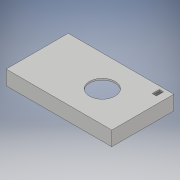
# Autodesk Inventor part: carrier_cmount
Saved by Autodesk Inventor 2018 (Build 220112000, 112)
## iProperties
Created: 2018-07-23
Part Number: carrier_cmount
Material: Generic
Document SubType Name: Modeling
Designer: matth
Density: 1 g/cm^3
Appearance: Default
Author: matth
Autodesk Inventor part; units mm, degrees
ref_plane "YZ Plane" through (0, 0, 0) normal (1, 0, 0) x (0, 1, 0)
ref_plane "XZ Plane" through (0, 0, 0) normal (0, 1, 0) x (-1, 0, 0)
ref_plane "XY Plane" through (0, 0, 0) normal (0, 0, 1) x (1, 0, 0)
sketch "Sketch1" plane through (0, 0, 0) normal (0, 0, 1) x (1, 0, 0)
  line L0 (-5.688, 3.2706) -> (94.312, 3.2706)
  line L1 (94.312, 3.2706) -> (94.312, -54.2294)
  line L2 (94.312, -54.2294) -> (-5.688, -54.2294)
  line L3 (-5.688, -54.2294) -> (-5.688, 3.2706)
  line L4 (95.812, 4.7706) -> (-7.188, 4.7706)
  line L5 (-7.188, 4.7706) -> (-7.188, -55.7294)
  line L6 (-7.188, -55.7294) -> (95.812, -55.7294)
  line L7 (95.812, -55.7294) -> (95.812, 4.7706)
  circle A0 centre (56.312, -25.4794) radius 12.5
  point P0 (0, 0)
  dimension "d0" = 100
  dimension "d1" = 57.5
  dimension "d2" = 1.5
  dimension "d3" = 25
  dimension "d4" = 38
  constraints: 16 end point, 4 parallel, 2 perpendicular, 1 centre point, 1 horizontal, 3 other
  measures "d0" distance of L1.end L2.end
  measures "d1" distance of L0.end L1.end
  measures "d2" distance between parallel lines of L0 L4
  measures "d3" diameter of A0
  measures "d4" distance from line of L1 A0.centre
extrude "Extrusion1" add sketch "Sketch1" along normal blind 1.5 contours L0 L1 L2 L3 | L7 L6 L5 L4
sketch "Sketch2" plane through (0, 0, 1.5) normal (0, 0, 1) x (1, 0, 0)
  line L0 (95.812, 4.7706) -> (-7.188, 4.7706) projected
  line L1 (-7.188, 4.7706) -> (-7.188, -55.7294) projected
  line L2 (-7.188, -55.7294) -> (95.812, -55.7294) projected
  line L3 (95.812, -55.7294) -> (95.812, 4.7706) projected
  line L4 (-5.688, 3.2706) -> (94.312, 3.2706)
  line L5 (94.312, 3.2706) -> (94.312, -54.2294)
  line L6 (94.312, -54.2294) -> (-5.688, -54.2294)
  line L7 (-5.688, -54.2294) -> (-5.688, 3.2706)
  point P0 (0, 0)
  dimension "d7" = 1.5
  constraints: 8 end point, 3 other
  measures "d7" distance between parallel lines of L0 L4
extrude "Extrusion2" add sketch "Sketch2" along normal blind 12.6
sketch "Sketch3" plane through (0, 0, 0) normal (0, 0, -1) x (-1, 0, 0)
  line L0 (-84.812, -45.7294) -> (-88.812, -45.7294)
  line L1 (-88.812, -45.7294) -> (-88.812, -52.7294)
  line L2 (-88.812, -52.7294) -> (-84.812, -52.7294)
  line L3 (-84.812, -52.7294) -> (-84.812, -45.7294)
  line L4 (7.188, -55.7294) -> (-95.812, -55.7294) projected
  line L5 (-95.812, -55.7294) -> (-95.812, 4.7706) projected
  point P0 (0, 0)
  dimension "d10" = 3
  dimension "d11" = 7
  dimension "d12" = 4
  dimension "d13" = 10
  constraints: 8 end point, 2 parallel, 1 horizontal, 1 perpendicular
  measures "d10" distance between parallel lines of L4 L2
  measures "d11" distance between parallel lines of L5 L1
  measures "d12" distance between parallel lines of L3 L1
  measures "d13" distance between parallel lines of L4 L0
extrude "Extrusion3" cut sketch "Sketch3" against normal up to next
sketch "Sketch4" plane through (-7.188, -55.7294, 0) normal (-1, 0, 0) x (0, 0, 1)
  line L0 (14.1, 60.5) -> (14.1, 0) projected
  line L1 (14.1, 48) -> (5.1, 48)
  line L2 (5.1, 48) -> (5.1, 33)
  line L3 (5.1, 33) -> (14.1, 33)
  line L4 (14.1, 33) -> (14.1, 48)
  line L5 (0, 60.5) -> (14.1, 60.5) projected
  line L6 (14.1, 11.5) -> (1.5, 11.5)
  line L7 (1.5, 11.5) -> (1.5, 22)
  line L8 (1.5, 22) -> (14.1, 22)
  line L9 (14.1, 22) -> (14.1, 11.5)
  point P0 (0, 55.7294)
  dimension "d16" = 9
  dimension "d18" = 27.5
  dimension "d19" = 12.5
  dimension "d20" = 12.6
  dimension "d21" = 49
  dimension "d22" = 38.5
  constraints: 16 end point, 4 parallel, 2 horizontal, 2 perpendicular, 2 point on line
  measures "d16" distance of L3.end L2.end
  measures "d18" distance between parallel lines of L3 L5
  measures "d19" distance between parallel lines of L5 L1
  measures "d20" distance of L8.end L7.end
  measures "d21" distance between parallel lines of L6 L5
  measures "d22" distance between parallel lines of L5 L8
extrude "Extrusion4" cut sketch "Sketch4" against normal up to surface (1.5 mm away)
sketch "Sketch5" plane through (0, 0, 1.5) normal (0, 0, 1) x (1, 0, 0)
  circle A0 centre (-2.938, -0.4794) radius 1.5
  circle A1 centre (91.562, -0.4794) radius 1.5
  circle A2 centre (-2.938, -50.4794) radius 1.5
  circle A3 centre (91.562, -50.4794) radius 1.5
  line L0 (-5.688, 3.2706) -> (94.312, 3.2706) projected
  line L1 (94.312, -54.2294) -> (-5.688, -54.2294) projected
  line L2 (94.312, 3.2706) -> (94.312, -54.2294) projected
  line L3 (-5.688, -54.2294) -> (-5.688, -44.2294) projected
  line L4 (-5.688, -7.7294) -> (-5.688, 3.2706) projected
  point P0 (0, 0)
  dimension "d25" = 3
  dimension "d26" = 3
  dimension "d27" = 3
  dimension "d28" = 3
  dimension "d31" = 3.75
  dimension "d32" = 3.75
  dimension "d33" = 3.75
  dimension "d34" = 2.75
  dimension "d35" = 2.75
  dimension "d36" = 2.75
  dimension "d37" = 3.75
  dimension "d39" = 2.75
  constraints: 4 centre point
  measures "d25" diameter of A0
  measures "d26" diameter of A1
  measures "d27" diameter of A2
  measures "d28" diameter of A3
  measures "d31" distance from line of L0 A0.centre
  measures "d32" distance from line of L0 A1.centre
  measures "d33" distance from line of L1 A3.centre
  measures "d34" distance from line of L2 A3.centre
  measures "d35" distance from line of L2 A1.centre
  measures "d36" distance from line of L3 A2.centre
  measures "d37" distance from line of L1 A2.centre
  measures "d39" distance from line of L4 A0.centre
extrude "Extrusion5" add sketch "Sketch5" along normal blind 12.6
sketch "Sketch6" plane through (0, 0, 1.5) normal (0, 0, 1) x (1, 0, 0)
  line L0 (-5.688, 3.2706) -> (-5.688, -33.7294) projected
  line L1 (-5.688, 3.2706) -> (0.312, 3.2706)
  line L2 (0.312, 3.2706) -> (0.312, -2.7294)
  line L3 (0.312, -2.7294) -> (-5.688, -2.7294)
  line L4 (-5.688, -2.7294) -> (-5.688, 3.2706)
  line L5 (94.312, 3.2706) -> (-5.688, 3.2706) projected
  line L6 (94.312, 3.2706) -> (88.312, 3.2706)
  line L7 (88.312, 3.2706) -> (88.312, -2.7294)
  line L8 (88.312, -2.7294) -> (94.312, -2.7294)
  line L9 (94.312, -2.7294) -> (94.312, 3.2706)
  line L10 (-5.688, -54.2294) -> (94.312, -54.2294) projected
  line L11 (88.812, -45.7294) -> (88.812, -52.7294) projected
  line L12 (94.312, -54.2294) -> (88.812, -54.2294)
  line L13 (88.812, -54.2294) -> (88.812, -47.9671)
  line L14 (88.812, -47.9671) -> (94.312, -47.9671)
  line L15 (94.312, -47.9671) -> (94.312, -54.2294)
  line L16 (-5.688, -54.2294) -> (0.312, -54.2294)
  line L17 (0.312, -54.2294) -> (0.312, -48.2294)
  line L18 (0.312, -48.2294) -> (-5.688, -48.2294)
  line L19 (-5.688, -48.2294) -> (-5.688, -54.2294)
  point P0 (0, 0)
  dimension "d42" = 6
  dimension "d43" = 6
  dimension "d44" = 6
  dimension "d45" = 6
  dimension "d46" = 6
  dimension "d47" = 6
  constraints: 32 end point, 8 parallel, 4 horizontal, 4 perpendicular, 3 point on line
  measures "d42" distance of L2.end L3.end
  measures "d43" distance of L1.end L2.end
  measures "d44" distance of L8.end L7.end
  measures "d45" distance of L7.end L6.end
  measures "d46" distance of L18.end L17.end
  measures "d47" distance of L17.end L16.end
extrude "Extrusion6" add sketch "Sketch6" along normal blind 10.6
body "Solid1"
